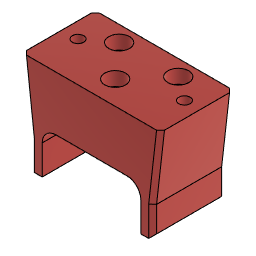
BF15 Mount (Autodesk Fusion 360 design; units mm, degrees)
Autodesk Fusion 360 part; units mm, degrees
note: some values were not read from the file. Set by a fixed rule: which sketch regions a step uses.
sketch "Sketch1" plane through (0, 0, 0) normal (0, 1, 0) x (1, 0, 0)
  line L0 (0, 0) -> (18, 0)
  line L1 (0, 0) -> (-18, 0)
  line L2 (25, 7) -> (25, 22)
  line L3 (-25, 7) -> (-25, 22)
  line L4 (25, 22) -> (31, 22)
  line L5 (-25, 22) -> (-31, 22)
  line L6 (0, 0) -> (0, -27.55) construction
  line L7 (0, -27.55) -> (35, -27.55)
  line L8 (0, -27.55) -> (-35, -27.55)
  line L9 (31, 22) -> (31, 7)
  line L10 (-31, 22) -> (-31, 7)
  line L11 (-35, -27.55) -> (-31, 7)
  line L12 (35, -27.55) -> (31, 7)
  arc A0 (-25, 7) -> (-18, 0) centre (-18, 7) ccw
  arc A1 (18, 0) -> (25, 7) centre (18, 7) ccw
  point P0 (25, 0)
  point P1 (-25, 0)
  dimension "d5" = 25
  dimension "d6" = 25
  dimension "d7" = 22
  dimension "d8" = 22
  dimension "d9" = 6
  dimension "d10" = 6
  dimension "d11" = 27.55
  dimension "d12" = 35
  dimension "d13" = 35
  dimension "d14" = 15
  dimension "d15" = 15
  dimension "d16" = 7
  dimension "d17" = 7
  constraint coincident L0.start L1.start
  constraint horizontal L0
  constraint parallel L0 L1
  constraint perpendicular L0 L2
  constraint perpendicular L1 L3
  constraint perpendicular L2 L4
  constraint perpendicular L3 L5
  constraint perpendicular L0 L6
  constraint perpendicular L6 L7
  constraint perpendicular L6 L8
  constraint perpendicular L4 L9
  constraint perpendicular L5 L10
  constraint coincident P1 L3
  constraint coincident P1 L1
  constraint tangent L3 A0
  constraint tangent L1 A0
  constraint coincident P0 L2
  constraint coincident P0 L0
  constraint tangent L2 A1
  constraint tangent L0 A1
  measures "d5" distance of L0.start P0
  measures "d6" distance of L0.start P1
  measures "d7" distance of P0 L2.end
  measures "d8" distance of P1 L3.end
  measures "d9" distance of L2.end L4.end
  measures "d10" distance of L3.end L5.end
  measures "d11" distance of L0.start L6.end
  measures "d12" distance of L6.end L7.end
  measures "d13" distance of L6.end L8.end
  measures "d14" distance of L4.end L9.end
  measures "d15" distance of L5.end L10.end
  measures "d16" radius of A0
  measures "d17" radius of A1
extrude "Extrude1" add sketch "Sketch1" along normal blind 37
sketch "Sketch2" plane through (0, 0, 27.55) normal (0, 0, 1) x (-1, 0, 0)
  line L0 (35, 0) -> (-35, 0)
  line L1 (-35, 0) -> (-35, -37)
  line L2 (-35, -37) -> (35, -37)
  line L3 (35, -37) -> (35, 0)
  line L4 (0, -37) -> (0, -29) construction
  line L5 (0, 0) -> (0, -12) construction
  line L6 (0, -29) -> (-15, -29) construction
  line L7 (0, -29) -> (15, -29) construction
  circle A0 centre (15, -29) radius 3.5
  circle A1 centre (15, -29) radius 5.25
  circle A2 centre (-15, -29) radius 3.5
  circle A3 centre (-15, -29) radius 5.25
  circle A4 centre (0, -12) radius 3.5
  circle A5 centre (0, -12) radius 5.25
  line L8 (-35, 0) -> (-27, 0) construction
  line L9 (-27, 0) -> (-27, -20.15) construction
  line L10 (-27, -20.15) -> (-35, -20.15) construction
  line L11 (-35, -20.15) -> (-35, 0) construction
  line L12 (35, 0) -> (27, 0) construction
  line L13 (27, 0) -> (27, -20.15) construction
  line L14 (27, -20.15) -> (35, -20.15) construction
  line L15 (35, -20.15) -> (35, 0) construction
  circle A6 centre (-27, -20.15) radius 2.9
  circle A7 centre (27, -20.15) radius 2.9
  dimension "d20" = 8
  dimension "d21" = 12
  dimension "d22" = 15
  dimension "d23" = 15
  dimension "d24" = 7
  dimension "d25" = 10.5
  dimension "d26" = 7
  dimension "d27" = 10.5
  dimension "d28" = 7
  dimension "d29" = 10.5
  dimension "d30" = 8
  dimension "d31" = 20.15
  dimension "d32" = 8
  dimension "d33" = 20.15
  dimension "d37" = 5.8
  dimension "d38" = 5.8
  constraint midpoint L2 L4.start
  constraint perpendicular L2 L4
  constraint coincident L5.start origin
  constraint perpendicular L0 L5
  constraint perpendicular L4 L6
  constraint perpendicular L4 L7
  constraint coincident L7.end A0.centre
  constraint concentric A0 A1
  constraint coincident L6.end A2.centre
  constraint coincident L5.end A4.centre
  constraint concentric A4 A5
  constraint horizontal L8
  constraint vertical L9
  constraint horizontal L10
  constraint vertical L11
  constraint coincident L0.end L1.start
  constraint horizontal L12
  constraint vertical L13
  constraint horizontal L14
  constraint vertical L15
  constraint coincident L0.start L3.end
  constraint coincident L9.end L10.start
  constraint coincident L13.end L14.start
  measures "d20" distance of L4.start L4.end
  measures "d21" distance of L5.start L5.end
  measures "d22" distance of L4.end L6.end
  measures "d23" distance of L4.end L7.end
  measures "d24" diameter of A0
  measures "d25" diameter of A1
  measures "d26" diameter of A2
  measures "d27" diameter of A3
  measures "d28" diameter of A4
  measures "d29" diameter of A5
  measures "d30" distance of L0.end L8.end
  measures "d31" distance of L0.end L10.end
  measures "d32" distance of L0.start L12.end
  measures "d33" distance of L0.start L14.end
  measures "d37" diameter of A6
  measures "d38" diameter of A7
extrude "Extrude4" cut sketch "Sketch2" against normal through all contours A0 | A2 | A4
extrude "Extrude3" cut sketch "Sketch2" against normal blind 7 contours A1 | A3 | A5
extrude "Extrude2" cut sketch "Sketch2" against normal up to surface (27.55 mm away) contours A6 | A7
chamfer "Chamfer1" distance 2 angle 45 8 edges at (33, 0, 10.275) (31, 0, -14.5) (-31, 0, -14.5) (-33, 0, 10.275) (-31, 37, -14.5) (-33, 37, 10.275) (33, 37, 10.275) (31, 37, -14.5)
chamfer "Chamfer2" distance 2 angle 45 2 edges at (-31, 18.5, -22) (31, 18.5, -22)
equation "steelRadius = 7 mm"
equation "steelNarrow = 50 mm"
equation "d5 = steelNarrow / 2"
equation "d6 = steelNarrow / 2"
equation "d16 = steelRadius"
equation "d17 = steelRadius"
